Autodesk Fusion 360 part; units mm, degrees
(part 2 of 2)
equation "d392 = Bearing_width / 2"
named bodies: "ball_38mm", "bearing", "A9800_orig", "A9800", "A9800_placement", "bearing2", "bearing (1)", "bearing3", "base_38mm", "bearing_holder", "bearing_holder (1)", "bearing_holder (2)", "Micro_holder_front", "Micro_holder_rear", "bottom", "kyria_mockup", "TOPA", "MIDDLEA_0", "MIDDLEBA", "MIDDLEBB", "MIDDLEBA (1)", "MIDDLEBB (1)", "MIDDLEA_1", "TEMP_PRINT", "TOPB_0", "TOPC_0", "PLATE_BOTTOM", "PLATE_MID", "PLATE_TOP", "ball_34mm", "base_34mm"
